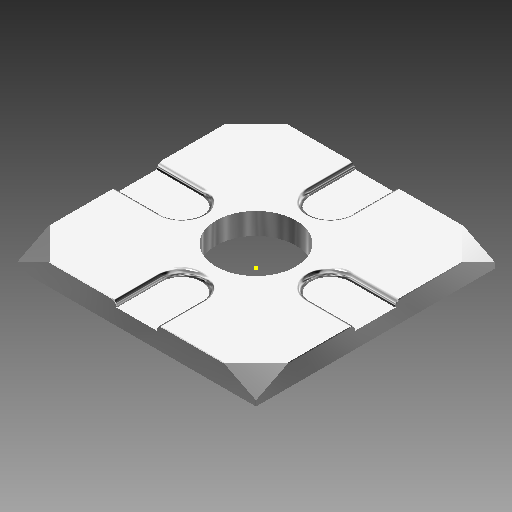
# Autodesk Inventor part: SSR-40 DA Big Plate
Saved by Autodesk Inventor 2019 (Build 230136000, 136)
## iProperties
Created: 2014-10-31
Part Number: SSR-40 DA Big Plate
Material: Nickel-Copper Alloy 400
Document SubType Name: Modeling
Designer: Tyler
Density: 8.83 g/cm^3
Appearance: Chrome - Polished
Author: Tyler
Autodesk Inventor part; units mm, degrees
ref_plane "YZ Plane" through (0, 0, 0) normal (1, 0, 0) x (0, 1, 0)
ref_plane "XZ Plane" through (0, 0, 0) normal (0, 1, 0) x (-1, 0, 0)
ref_plane "XY Plane" through (0, 0, 0) normal (0, 0, 1) x (1, 0, 0)
sketch "Sketch1" plane through (0, 0, 0) normal (0, 1, 0) x (-1, 0, 0)
  line L0 (5.8928, 5.8928) -> (-5.8928, 5.8928)
  line L1 (-5.8928, 5.8928) -> (-5.8928, -5.8928)
  line L2 (-5.8928, -5.8928) -> (5.8928, -5.8928)
  line L3 (5.8928, -5.8928) -> (5.8928, 5.8928)
  point P0 (0, 0)
  point P1 (5.8928, 0)
  point P2 (0, -5.8928)
  dimension "d0" = 11.7856
  constraints: 8 end point, 2 midpoint, 2 parallel, 2 perpendicular, 1 horizontal, 1 horizontal alignment, 1 vertical alignment
  measures "d0" distance of L2.end L1.end
extrude "Extrusion1" add sketch "Sketch1" along normal blind 1.0668
sketch "Sketch2" plane through (0, 1.0668, 0) normal (0, 1, 0) x (1, 0, 0)
  line L0 (3.6703, -0.9779) -> (5.8928, -0.9779)
  line L1 (5.8928, -0.9779) -> (5.8928, 0.9779)
  line L2 (5.8928, 0.9779) -> (3.6703, 0.9779)
  line L3 (2.6924, 0) -> (2.6924, 0)
  line L4 (5.8928, -5.8928) -> (5.8928, 5.8928) projected
  arc A0 (3.6703, 0.9779) -> (2.6924, 0) centre (3.6703, 0) ccw
  arc A1 (2.6924, 0) -> (3.6703, -0.9779) centre (3.6703, 0) ccw
  line L5 (-0.9779, -5.8928) -> (0.9779, -5.8928)
  line L6 (0.9779, -5.8928) -> (0.9779, -3.6703)
  line L7 (0, -2.6924) -> (0, -2.6924)
  line L8 (-0.9779, -3.6703) -> (-0.9779, -5.8928)
  arc A2 (0.9779, -3.6703) -> (0, -2.6924) centre (0, -3.6703) ccw
  arc A3 (0, -2.6924) -> (-0.9779, -3.6703) centre (0, -3.6703) ccw
  line L9 (-5.8928, 5.8928) -> (-5.8928, -5.8928) projected
  line L10 (-5.8928, -0.9779) -> (-3.6703, -0.9779)
  line L11 (-2.6924, 0) -> (-2.6924, 0)
  line L12 (-3.6703, 0.9779) -> (-5.8928, 0.9779)
  line L13 (-5.8928, 0.9779) -> (-5.8928, -0.9779)
  arc A4 (-3.6703, -0.9779) -> (-2.6924, 0) centre (-3.6703, 0) ccw
  arc A5 (-2.6924, 0) -> (-3.6703, 0.9779) centre (-3.6703, 0) ccw
  line L14 (5.8928, 5.8928) -> (-5.8928, 5.8928) projected
  line L15 (-0.9779, 5.8928) -> (0.9779, 5.8928)
  line L16 (0.9779, 5.8928) -> (0.9779, 3.6703)
  line L17 (0, 2.6924) -> (0, 2.6924)
  line L18 (-0.9779, 3.6703) -> (-0.9779, 5.8928)
  arc A6 (-0.9779, 3.6703) -> (0, 2.6924) centre (0, 3.6703) ccw
  arc A7 (0, 2.6924) -> (0.9779, 3.6703) centre (0, 3.6703) ccw
  point P0 (0, 0)
  point P1 (2.6924, 0.9779)
  point P2 (2.6924, 0)
  point P3 (5.8928, 0)
  point P4 (5.8928, 0)
  point P5 (0.9779, -2.6924)
  point P6 (-0.9779, -2.6924)
  point P7 (0, -2.6924)
  point P8 (-2.6924, 0.9779)
  point P9 (-5.8928, 0)
  point P10 (-5.8928, 0)
  point P11 (0.9779, 2.6924)
  point P12 (0, 5.8928)
  point P13 (0, 5.8928)
  dimension "d3" = 3.2004
  dimension "d4" = 1.9558
  dimension "d5" = 0.9779
  dimension "d6" = 1.9558
  dimension "d7" = 3.2004
  dimension "d8" = 0.9779
  dimension "d9" = 3.2004
  dimension "d10" = 0.9779
  dimension "d11" = 3.2004
  dimension "d12" = 0.9779
  constraints: 32 end point, 16 point on circle, 16 tangent, 12 point on line, 8 centre point, 8 midpoint, 8 parallel, 4 concentric, 4 horizontal, 4 perpendicular, 3 horizontal alignment, 2 vertical alignment, 1 coincident
  measures "d3" distance of point (2.692, 0.978) L1.end
  measures "d4" distance of L1.end L0.end
  measures "d5" radius of A0
  measures "d6" distance of point (-0.978, -2.692) point (0.978, -2.692)
  measures "d7" distance of point (0.978, -2.692) L5.end
  measures "d8" radius of A2
  measures "d9" distance of L12.end point (-2.692, 0.978)
  measures "d10" radius of A4
  measures "d11" distance of L15.end point (0.978, 2.692)
  measures "d12" radius of A6
extrude "Extrusion2" cut sketch "Sketch2" against normal blind 0.2794
fillet "Fillet1" radius 0.2794 12 edges at (-4.7816, 1.0668, 0.9779) (-4.7816, 1.0668, -0.9779) (-2.6924, 1.0668, 0) (0, 1.0668, -2.6924) (0.9779, 1.0668, -4.7816) (-0.9779, 1.0668, -4.7816) (2.6924, 1.0668, 0) (4.7816, 1.0668, 0.9779) (4.7816, 1.0668, -0.9779) (0, 1.0668, 2.6924) (-0.9779, 1.0668, 4.7816) (0.9779, 1.0668, 4.7816)
sketch "Sketch3" plane through (0, 0, 0) normal (0, -1, 0) x (1, 0, 0)
  point P0 (0, 0)
sketch "Sketch4" plane through (0, 1.0668, 0) normal (0, 1, 0) x (1, 0, 0)
  circle A0 centre (0, 0) radius 1.9685
  dimension "d16" = 3.937
  constraints: 1 centre point, 1 coincident
  measures "d16" diameter of A0
extrude "Extrusion3" cut sketch "Sketch4" against normal through all
chamfer "Chamfer1" distance 0.0254 angle 45 24 edges at (5.8928, 1.0668, 3.575) (5.8928, 0.7875, 0.9779) (5.8928, 0.985, 1.0597) (3.575, 1.0668, 5.8928) (1.0597, 0.985, 5.8928) (0.9779, 0.7875, 5.8928) (5.8928, 1.0668, -3.575) (5.8928, 0.985, -1.0597) (5.8928, 0.7875, -0.9779) (3.575, 1.0668, -5.8928) (0.9779, 0.7875, -5.8928) (1.0597, 0.985, -5.8928) (-3.575, 1.0668, -5.8928) (-1.0597, 0.985, -5.8928) (-0.9779, 0.7875, -5.8928) (-5.8928, 1.0668, -3.575) (-5.8928, 0.7875, -0.9779) (-5.8928, 0.985, -1.0597) (-5.8928, 1.0668, 3.575) (-5.8928, 0.985, 1.0597) (-5.8928, 0.7875, 0.9779) (-3.575, 1.0668, 5.8928) (-0.9779, 0.7875, 5.8928) (-1.0597, 0.985, 5.8928)
chamfer "Chamfer2" distance 1.27 angle 45 4 edges at (5.8801, 1.0541, 5.8801) (5.8801, 1.0541, -5.8801) (-5.8801, 1.0541, -5.8801) (-5.8801, 1.0541, 5.8801)
fillet "Fillet2" radius 0.0254 4 edges at (-5.8928, 0.1318, 5.8928) (5.8928, 0.1318, 5.8928) (5.8928, 0.1318, -5.8928) (-5.8928, 0.1318, -5.8928)
body "Solid1"
